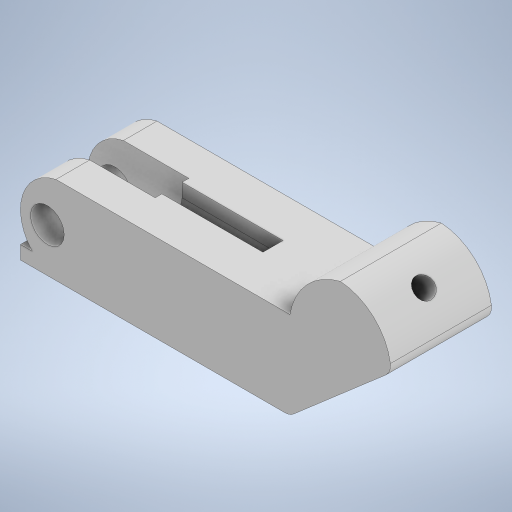
# Autodesk Inventor part: ProjEnAble_Finger
Saved by Autodesk Inventor 2023 (Build 270158000, 158)
## iProperties
Created: 2023-01-11
Part Number: ProjEnAble_Finger
Material: Generic
Document SubType Name: Modeling
Designer: jeron
Density: 1 g/cm^3
Appearance: Default
Author: jeron
Autodesk Inventor part; units mm, degrees
ref_plane "YZ Plane" through (0, 0, 0) normal (1, 0, 0) x (0, 1, 0)
sketch "Sketch1" plane through (0, 0, 0) normal (0, 0, 1) x (1, 0, 0)
  line L0 (0, 0) -> (39.2539, 0)
  line L1 (40, 13) -> (0, 13)
  line L2 (0, 13) -> (0, 0)
  circle A0 centre (4, 6.5) radius 4
  circle A1 centre (4, 6.5) radius 2.5
  line L3 (8, 13) -> (8, 0)
  arc A2 (5.2813, 13) -> (1.7572, 2) centre (6.6406, 6.5) ccw
  line L4 (40, 0) -> (55, 0)
  line L5 (55, 0) -> (55, 13)
  arc A3 (47.5, 21) -> (40, 13) centre (49.851, 11.2803) ccw
  line L6 (54.25, 12.35) -> (40.5638, 0.4886)
  arc A4 (54.9201, 14.1433) -> (47.5, 21) centre (47, 13.0156) ccw
  arc A5 (39.2539, 0) -> (40.5638, 0.4886) centre (39.2539, 2) ccw
  arc A6 (54.25, 12.35) -> (54.9201, 14.1433) centre (52.9401, 13.8614) ccw
  line L7 (8, 0) -> (8, 2)
  line L8 (8, 2) -> (-2, 2)
  line L9 (-2, 2) -> (-2, 0)
  line L10 (-2, 0) -> (8, 0)
  point P0 (0, 6.5)
  point P1 (0, 2)
  dimension "d2" = 8
  dimension "d0" = 40
  dimension "d3" = 5
  dimension "d4" = 15
  dimension "d5" = 13
  dimension "d7" = 10
  dimension "d8" = 8
  dimension "d9" = 2
  dimension "d10" = 2
  dimension "d11" = 10
  constraints: 22 end point, 12 point on circle, 8 point on line, 6 centre point, 4 perpendicular, 4 tangent, 2 horizontal, 1 coincident, 1 collinear, 1 equal radius, 1 horizontal alignment, 1 midpoint, 1 parallel, 2 other
  measures "d0" distance of L1.end L1.start
  measures "d3" diameter of A1
  measures "d4" distance of L4.start L4.end
  measures "d5" distance of L4.end L5.end
  measures "d7" radius of A3
  measures "d8" radius of A4
  measures "d9" radius of A5
  measures "d10" distance of L3.end L7.end
  measures "d11" distance of L7.end L8.end
extrude "Extrusion1" add sketch "Sketch1" along normal blind 15 contours L2 L8 L3 L0 | L3 L1 A3 A4 A6 L6 A5 L0 | L8 A2 A0 L3 | A2 L1 L3 A0 | A0
ref_plane "Work Plane1" through (5.2813, 23, 0) normal (0, 1, 0) x (1, 0, 0)
sketch "Sketch2" plane through (5.2813, 23, 0) normal (0, 1, 0) x (1, 0, 0)
  line L0 (-5.2813, 0) -> (-5.2813, -15) projected
  line L1 (-5.2813, -7.5) -> (-5.2813, -5)
  line L2 (-5.2813, -7.5) -> (-5.2813, -10)
  line L3 (-5.2813, -5) -> (9.7187, -5)
  line L4 (-5.2813, -10) -> (9.7187, -10)
  line L5 (9.7187, -10) -> (9.7187, -5)
  line L6 (9.7187, -7.5) -> (9.7187, -6)
  line L7 (9.7187, -7.5) -> (9.7187, -9)
  line L8 (9.7187, -9) -> (24.7188, -9)
  line L9 (24.7188, -9) -> (24.7188, -6)
  line L10 (24.7188, -6) -> (9.7187, -6)
  dimension "d15" = 2.5
  dimension "d16" = 2.5
  dimension "d17" = 15
  dimension "d18" = 15
  dimension "d19" = 1.5
  dimension "d20" = 1.5
  dimension "d21" = 15
  constraints: 20 end point, 4 perpendicular, 4 point on line, 2 midpoint, 1 horizontal
  measures "d15" distance of L1.start L1.end
  measures "d16" distance of L1.start L2.end
  measures "d17" distance of L1.end L3.end
  measures "d18" distance of L2.end L4.end
  measures "d19" distance of L6.start L6.end
  measures "d20" distance of L6.start L7.end
  measures "d21" distance of L7.end L8.end
extrude "Extrusion2" cut sketch "Sketch2" against normal through all contours L3 L5 L4 L0
sketch "Sketch3" plane through (15, 0, 5) normal (-1, 0, 0) x (0, 0, 1)
  line L0 (0, 13) -> (5, 13) projected
  circle A0 centre (2.5, 11) radius 1.5
  circle A1 centre (2.5, 2) radius 1.5
  line L1 (5, 0) -> (0, 0) projected
  point P0 (-5, 0)
  point P1 (2.5, 0)
  dimension "d25" = 3
  dimension "d27" = 3
  constraints: 2 centre point, 1 midpoint
  measures "d25" diameter of A0
  measures "d27" diameter of A1
extrude "Extrusion3" cut sketch "Sketch3" against normal through all contours A1
extrude "Extrusion4" cut sketch "Sketch3" against normal blind 26 contours A0
extrude "Extrusion5" cut sketch "Sketch2" against normal blind 12 contours L10 L9 L8 L5
ref_plane "Work Plane2" through (52.4294, 18.8912, 0) normal (0.678674, 0.7344396, 0) x (-0.7344396, 0.678674, 0)
sketch "Sketch4" plane through (52.4294, 18.8912, 0) normal (0.678674, 0.7344396, 0) x (-0.7344396, 0.678674, 0)
  circle A0 centre (0, 7.5) radius 1.5
  point P0 (25.6853, 0)
  point P1 (5.0516, 15)
  point P2 (-5.0516, 15)
  dimension "d34" = 3
  constraints: 1 centre point
  measures "d34" diameter of A0
loft "Loft1" cut profiles "Sketch4" section 2 edges at (41, 11, 6)
body "Solid1"
